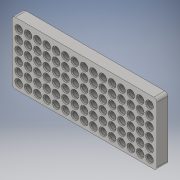
# Autodesk Inventor part: chassis_plate
Saved by Autodesk Inventor 2016 (Build 200138000, 138)
## iProperties
Created: 2016-02-13
Part Number: chassis_plate
Material: Generic
Document SubType Name: Modeling
Designer: jforce
Density: 1 g/cm^3
Appearance: Default
Author: jforce
## iProperties of the stored document chassis_plate_3DPrint.ipt
Created: 2016-02-15
Part Number: chassis_plate_3DPrint
Material: Generic
Document SubType Name: Modeling
Designer: jforce
Density: 1 g/cm^3
Appearance: Default
Author: jforce
Autodesk Inventor part; units mm, degrees
ref_plane "YZ Plane" through (0, 0, 0) normal (1, 0, 0) x (0, 1, 0)
ref_plane "XZ Plane" through (0, 0, 0) normal (0, 1, 0) x (-1, 0, 0)
ref_plane "XY Plane" through (0, 0, 0) normal (0, 0, 1) x (1, 0, 0)
sketch "Sketch1" plane through (0, 0, 0) normal (0, 0, 1) x (1, 0, 0)
  line L0 (2, 0) -> (91, 0)
  line L1 (93, 2) -> (93, 38)
  line L2 (91, 40) -> (2, 40)
  line L3 (0, 38) -> (0, 2)
  arc A0 (93, 38) -> (91, 40) centre (91, 38) ccw
  arc A1 (2, 40) -> (0, 38) centre (2, 38) ccw
  arc A2 (0, 2) -> (2, 0) centre (2, 2) ccw
  arc A3 (91, 0) -> (93, 2) centre (91, 2) ccw
  point P0 (0, 0)
  point P1 (93, 40)
  point P2 (93, 0)
  point P3 (0, 40)
  dimension "d0" = 93
  dimension "d1" = 40
  dimension "d2" = 2
  constraints: 8 end point, 8 point on circle, 8 point on line, 8 tangent, 4 centre point, 3 equal radius, 2 parallel, 1 horizontal, 1 perpendicular
  measures "d0" distance of point (93, 40) point (0, 40)
  measures "d1" distance of point (93, 0) point (93, 40)
  measures "d2" radius of A0
extrude "Extrusion1" add sketch "Sketch1" along normal blind 7
sketch "Sketch2" plane through (0, 0, 7) normal (0, 0, 1) x (1, 0, 0)
  point P0 (0, 0)
  point P1 (4.2467, 4.3978)
hole "Hole1" at (4.2467, 4.3978, 7) direction (0, 0, -1) diameter 4 depth 7 tip angle 118 counterbore diameter 5 counterbore depth 0.85
sketch "Sketch3" plane through (0, 0, 0) normal (0, 0, -1) x (-1, 0, 0)
  circle A0 centre (-4.2467, 4.3978) radius 2 projected
  circle A1 centre (-4.2467, 4.3978) radius 2.5
  point P0 (0, 0)
  dimension "d12" = 5
  constraints: 1 centre point, 1 coincident
  measures "d12" diameter of A1
extrude "Extrusion2" cut sketch "Sketch3" against normal blind 0.85
pattern_linear "Rectangular Pattern1" count 15 spacing 6 along (1, 0, 0) count 6 spacing 6 along (0, 1, 0) of "Hole1", "Extrusion2"
body "Solid1"
